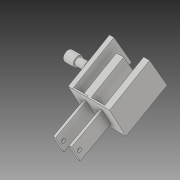
# Autodesk Inventor part: grip
Saved by Autodesk Inventor 2017 (Build 210142000, 142)
## iProperties
Created: 2021-04-21
Part Number: grip
Material: Generic
Document SubType Name: Modeling
Designer: Anthony
Density: 1 g/cm^3
Appearance: Default
Author: Anthony
Autodesk Inventor part; units mm, degrees
sketch "Sketch1" plane through (0, 0, 0) normal (1, 0, 0) x (0, 1, 0)
  line L0 (15, -38) -> (-51, -38)
  line L1 (-51, -38) -> (-51, -56)
  line L2 (-51, -56) -> (15, -56)
  line L3 (15, -38) -> (15, -56)
  arc A0 (29.5, -43.2058) -> (20.5, -58.7942) centre (25, -51) ccw
  arc A1 (33.0623, -37.0358) -> (16.9377, -64.9642) centre (25, -51) ccw
  line L4 (29.5, -43.2058) -> (39.0263, -48.7058)
  line L5 (20.5, -58.7942) -> (30.0263, -64.2942)
  line L6 (16.9377, -64.9642) -> (26.464, -70.4642)
  line L7 (33.0623, -37.0358) -> (42.5885, -42.5358)
  line L8 (42.5885, -42.5358) -> (39.0263, -48.7058)
  line L9 (30.0263, -64.2942) -> (26.464, -70.4642)
  line L10 (-51, -38) -> (-79, -38)
  line L11 (-79, -38) -> (-79, -56)
  line L12 (-51, -56) -> (-79, -56)
  dimension "d1" = 18
  constraints: 26 end point, 5 perpendicular, 4 point on circle, 3 tangent, 2 centre point, 2 horizontal, 1 coincident, 1 vertical
  measures "d1" diameter of A0
extrude "Extrusion1" add sketch "Sketch1" along normal blind 10 contours L3 A1 L2 L1 L0 | A1 L7 L8 L4 A0 L5 L9 L6 L2 L3 | L3 L2 A1
thicken "Thicken1" operation add thickness 5 both sides no extend neighbours yes toward (0, 0.8660254, -0.5) faces at (3.3333, 28.8389, -66.3509)
thicken "Thicken2" operation add thickness 5 both sides no extend neighbours yes toward (0, 0.8660254, -0.5) faces at (3.3333, 41.4011, -44.5924)
thicken "Thicken3" operation add thickness 200 both sides no extend neighbours yes toward (0, -1, 0) faces at (3.3333, -51, -44)
thicken "Thicken4" operation add thickness 30 both sides no extend neighbours yes toward (-1, 0, 0) faces at (0, -75.4432, -44)
sketch "Sketch2" plane through (10, 0, 0) normal (1, 0, 0) x (0, 0, -1)
  arc A0 (37.0358, 33.0623) -> (38.3509, 15) centre (51, 25) ccw projected
  line L0 (56, 10) -> (38.3509, 15)
  line L1 (38.3509, 15) -> (23, -17)
  line L2 (23, -17) -> (9, -332)
  line L3 (9, -332) -> (100, -328)
  line L4 (100, -328) -> (71, -47)
  line L5 (71, -47) -> (56, 10)
  point P0 (0, 0)
  constraints: 12 end point
extrude "Extrusion2" cut sketch "Sketch2" against normal blind 100
sketch "Sketch3" plane through (10, 0, 0) normal (1, 0, 0) x (0, 0, -1)
  line L0 (56, 10) -> (152, -151)
  line L1 (152, -151) -> (131, -151)
  line L2 (38.3509, 15) -> (56, 10) projected
  line L3 (131, -151) -> (38.3509, 15)
  point P0 (0, 0)
  constraints: 6 end point, 1 horizontal
extrude "Extrusion3" add sketch "Sketch3" against normal blind 40
thicken "Thicken5" operation add thickness 100 both sides no extend neighbours yes toward (0, -1, 0) faces at (-3.3333, -151, -145)
sketch "Sketch4" plane through (10, 0, 0) normal (1, 0, 0) x (0, 0, -1)
  line L0 (29, -65) -> (197, -65)
  line L1 (197, -65) -> (243, -262)
  line L2 (243, -262) -> (173, -278.3452)
  line L3 (173, -278.3452) -> (29, -65)
  point P0 (0, 0)
  constraints: 8 end point, 1 horizontal, 1 perpendicular
extrude "Extrusion4" cut sketch "Sketch4" against normal blind 40
thicken "Thicken6" operation add thickness 40 both sides no extend neighbours yes toward (1, 0, 0) faces at (10, 14.7562, -38.117)
thicken "Thicken7" operation add thickness 5 both sides no extend neighbours yes toward (0, -0.5, -0.8660254) faces at (-16.6667, 26.1753, -70.2976) (-3.3333, 10.1872, -57.3703) (-3.3333, -15.1835, -71.0162)
ref_plane "Work Plane1" through (10, -65, -83.0011) normal (1, 0, 0) x (0, 0, -1)
sketch "Sketch6" plane through (10, -65, -83.0011) normal (1, 0, 0) x (0, 0, -1)
  line L0 (23.5408, 0) -> (0, 0) projected
  line L1 (23.5408, 0) -> (65, -73)
  line L2 (65, -73) -> (86.5815, -111)
  line L3 (0, 0) -> (-44.6502, 80) projected
  line L4 (0, 0) -> (59, -111)
  line L5 (59, -111) -> (86.5815, -111)
  point P0 (-83.0011, 65)
  constraints: 8 end point, 1 horizontal, 1 point on line
extrude "Extrusion6" add sketch "Sketch6" along normal mid plane 40
thicken "Thicken8" operation add thickness 100 both sides no extend neighbours yes toward (0, -1, 0) faces at (3.3333, -176, -151.1949)
thicken "Thicken9" operation add thickness 20 both sides no extend neighbours yes toward (0, 0.8660254, -0.5) faces at (-16.6667, 45.7312, -47.0924)
thicken "Thicken10" operation add thickness 20 both sides no extend neighbours yes toward (0, 0.8660254, -0.5) faces at (-3.3333, 32.3357, -70.2943)
sketch "Sketch7" plane through (30, -65, -83.0011) normal (1, 0, 0) x (0, 0, -1)
  line L0 (112.1532, -211) -> (143.3749, -211) projected
  line L1 (23.5408, 0) -> (143.3749, -211) projected
  line L2 (143.3749, -211) -> (130, -187.4499)
  line L3 (130, -187.4499) -> (99.6355, -187.4499)
  line L4 (0, 0) -> (112.1532, -211) projected
  line L5 (112.1532, -211) -> (99.6355, -187.4499)
  point P0 (-83.0011, 65)
  constraints: 6 end point, 2 point on line, 1 collinear, 1 horizontal
extrude "Extrusion7" add sketch "Sketch7" against normal blind 400
thicken "Thicken12" operation add thickness 65 both sides no extend neighbours yes toward (1, 0, 0) faces at (-370, -268.15, -211.5104)
sketch "Sketch8" plane through (-305, -276, -226.376) normal (-1, 0, 0) x (0, 0, 1)
  line L0 (43.7393, 23.5501) -> (13.3749, 23.5501) projected
  line L1 (43.7393, 23.5501) -> (20.991, 36.7127)
  line L2 (13.3749, 23.5501) -> (43.7393, 23.5501) projected
  line L3 (20.991, 36.7127) -> (13.3749, 23.5501)
  point P0 (226.376, 276)
  constraints: 4 end point, 1 perpendicular
extrude "Extrusion8" add sketch "Sketch8" against normal blind 300
sketch "Sketch9" plane through (-305, -239.2873, -205.385) normal (0, 0.8655505, 0.5008216) x (1, 0, 0)
  line L0 (0, -0.2177) -> (0, -27.2417) projected
  line L1 (0, -0.2177) -> (0, -27.2417)
  line L2 (0, -27.2417) -> (29, -27.2417)
  line L3 (0, -27.2417) -> (335, -27.2417) projected
  line L4 (0, -0.2177) -> (29, -0.2177)
  line L5 (0, -0.2177) -> (335, -0.2177) projected
  line L6 (29, -27.2417) -> (29, -0.2177)
  point P0 (305, -57.9308)
  constraints: 8 end point, 2 point on line, 1 perpendicular, 1 vertical
extrude "Extrusion9" add sketch "Sketch9" along normal blind 70
thicken "Thicken13" operation add thickness 15 both sides no extend neighbours yes toward (0, -0.8655505, -0.5008216) faces at (-295.3333, -187.8307, -154.5452)
thicken "Thicken14" operation add thickness 7 both sides no extend neighbours yes toward (0, -0.8655505, -0.5008216) faces at (-295.3333, -200.8139, -162.0576)
sketch "Sketch10" plane through (-276, -239.3964, -205.1965) normal (0, 0.5008216, -0.8655505) x (-1, 0, 0)
  line L0 (0, 48) -> (29, 48) projected
  line L1 (0, 48) -> (-35, 48)
  line L2 (-35, 48) -> (-35, 81)
  line L3 (-35, 81) -> (-35, 106)
  line L4 (29, 48) -> (29, 121)
  line L5 (-35, 106) -> (-35, 138)
  line L6 (-35, 138) -> (-45, 138)
  line L7 (-45, 138) -> (-45, 41)
  line L8 (-45, 41) -> (29, 41)
  line L9 (29, 0) -> (29, 48) projected
  line L10 (29, 41) -> (29, 48)
  line L11 (29, 48) -> (29, 41)
  line L12 (29, 121) -> (29, 141)
  line L13 (29, 141) -> (38, 141)
  line L14 (38, 141) -> (38, 41)
  line L15 (38, 41) -> (29, 41)
  line L16 (29, 81) -> (0, 81)
  line L17 (0, 81) -> (0, 48)
  point P0 (-276, 309.9765)
  dimension "d49" = 35
  constraints: 32 end point, 8 perpendicular, 4 vertical, 2 horizontal, 2 point on line, 1 collinear
  measures "d49" distance of L0.start L1.end
extrude "Extrusion10" add sketch "Sketch10" along normal blind 70 contours L0 L9 L8 L7 L6 L5 L3 L2 L1 | L4 L12 L13 L14 L15 L9
sketch "Sketch12" plane through (-276, -204.3389, -265.785) normal (0, 0.5008216, -0.8655505) x (-1, 0, 0)
  line L0 (29, 48) -> (0, 48) projected
  line L1 (14.5, 48) -> (14.5, 123)
  line L2 (14.5, 123) -> (-8, 123)
  line L3 (-8, 123) -> (-8, 48)
  line L4 (-8, 48) -> (14.5, 48)
  point P0 (-276, 309.9765)
  constraints: 8 end point, 2 perpendicular, 1 collinear, 1 midpoint, 1 vertical
extrude "Extrusion11" add sketch "Sketch12" against normal blind 70
thicken "Thicken15" operation add thickness 2 both sides no extend neighbours yes toward (-1, 0, 0) faces at (-268, -142.8866, -176.3122)
thicken "Thicken16" operation add thickness 2 both sides no extend neighbours yes toward (1, 0, 0) faces at (-290.5, -142.8866, -176.3122)
thicken "Thicken17" operation add thickness 4 both sides no extend neighbours yes toward (1, 0, 0) faces at (-288.5, -142.8866, -176.3122)
thicken "Thicken18" operation add thickness 2 both sides no extend neighbours yes toward (-1, 0, 0) faces at (-241, -160.1976, -186.3286)
ref_plane "Work Plane2" through (-137.5, -65, -83.0011) normal (1, 0, 0) x (0, 0, -1)
sketch "Sketch13" plane through (-137.5, -65, -83.0011) normal (1, 0, 0) x (0, 0, -1)
  line L0 (143.3749, -211) -> (112.1532, -211) projected
  line L1 (130, -187.4499) -> (143.3749, -211) projected
  line L2 (143.3749, -211) -> (14, -211)
  line L3 (14, -211) -> (14, -187.4499)
  line L4 (14, -187.4499) -> (130, -187.4499)
  point P0 (-83.0011, 65)
  constraints: 6 end point, 2 perpendicular, 1 point on line
extrude "Extrusion12" add sketch "Sketch13" along normal mid plane 30
thicken "Thicken19" operation add thickness 150 both sides no extend neighbours yes toward (0, 0, 1) faces at (-142.5, -260.3, -97.0011)
thicken "Thicken20" operation add thickness 20 both sides no extend neighbours yes toward (0, 0, -1) faces at (-142.5, -260.3, 52.9989)
sketch "Sketch14" plane through (-152.5, -276, 32.9989) normal (0, 0, 1) x (1, 0, 0)
  line L0 (30, 23.5501) -> (30, 0) projected
  line L1 (0, 23.5501) -> (30, 23.5501) projected
  line L2 (0, 0) -> (30, 0) projected
  line L3 (0, 0) -> (0, 23.5501) projected
  circle A0 centre (15, 11.775) radius 8
  point P0 (152.5, 276)
  constraints: 1 centre point
extrude "Extrusion13" add sketch "Sketch14" along normal blind 70 contours A0
thicken "Thicken21" operation add thickness 30 both sides no extend neighbours yes toward (0, 0, -1) faces at (-134.9108, -264.8631, 102.9989)
sketch "Sketch15" plane through (-122.5, -65, -83.0011) normal (1, 0, 0) x (0, 0, -1)
  arc A0 (-202, -264) -> (-180, -132) centre (-216.7127, -193.7146) ccw
  arc A1 (-204.0725, -254.0995) -> (-185.1714, -140.6932) centre (-216.7127, -193.7146) ccw
  arc A2 (-200.0254, -273.433) -> (-175.0728, -123.7173) centre (-216.7127, -193.7146) ccw
  line L0 (-175.0728, -123.7173) -> (-185.1714, -140.6932)
  line L1 (-204.0725, -254.0995) -> (-200.0254, -273.433)
  point P0 (-83.0011, 65)
  constraints: 6 point on circle, 4 end point, 3 centre point
extrude "Extrusion14" add sketch "Sketch15" against normal blind 30
sketch "Sketch16" plane through (-122.5, -65, -83.0011) normal (1, 0, 0) x (0, 0, -1)
  point P0 (-83.0011, 65)
ref_plane "Work Plane3" through (-137.5, -65, -83.0011) normal (1, 0, 0) x (0, 0, -1)
sketch "Sketch17" plane through (-137.5, -65, -83.0011) normal (1, 0, 0) x (0, 0, -1)
  arc A0 (-204.0725, -254.0995) -> (-185.1714, -140.6932) centre (-216.7127, -193.7146) ccw projected
  arc A1 (-200.5833, -270.7677) -> (-176.465, -126.0576) centre (-216.7127, -193.7146) ccw
  line L0 (-176.465, -126.0576) -> (-223, -140.6932)
  line L1 (-223, -140.6932) -> (-219, -249)
  line L2 (-219, -249) -> (-200.5833, -270.7677)
  point P0 (-83.0011, 65)
  constraints: 6 end point, 2 point on circle, 1 centre point
extrude "Extrusion15" cut sketch "Sketch17" against normal blind 14
sketch "Sketch18" plane through (-122.5, -65, -83.0011) normal (1, 0, 0) x (0, 0, -1)
  point P0 (-83.0011, 65)
ref_plane "Work Plane4" through (-124.5, -65, -83.0011) normal (1, 0, 0) x (0, 0, -1)
sketch "Sketch19" plane through (-124.5, -65, -83.0011) normal (1, 0, 0) x (0, 0, -1)
  arc A0 (-200.0254, -273.433) -> (-175.0728, -123.7173) centre (-216.7127, -193.7146) ccw projected
  arc A1 (-200.6398, -270.4982) -> (-176.6058, -126.2942) centre (-216.7127, -193.7146) ccw
  line L0 (-176.6058, -126.2942) -> (-213.3412, -154.8678)
  line L1 (-213.3412, -154.8678) -> (-216.7127, -283)
  line L2 (-216.7127, -283) -> (-200.6398, -270.4982)
  point P0 (-83.0011, 65)
  constraints: 6 end point, 2 point on circle, 1 centre point, 1 parallel
extrude "Extrusion16" cut sketch "Sketch19" against normal blind 14
thicken "Thicken22" operation add thickness 150 both sides no extend neighbours yes toward (1, 0, 0) faces at (-122.5, -268.15, -114.9306)
thicken "Thicken23" operation add thickness 150 both sides no extend neighbours yes toward (1, 0, 0) faces at (-152.5, -268.15, -114.9306)
thicken "Thicken24" operation add thickness 150 both sides no extend neighbours yes toward (1, 0, 0) faces at (-122.5, -266.9722, 59.5019)
thicken "Thicken25" operation add thickness 150 both sides no extend neighbours yes toward (1, 0, 0) faces at (-152.5, -266.9722, 59.5019)
sketch "Sketch20" plane through (-137.5, -264.225, 32.9989) normal (0, 0, -1) x (-1, 0, 0)
  circle A0 centre (0, 0) radius 10.0499
  point P0 (-137.5, 264.225)
  constraints: 1 centre point, 1 other
extrude "Extrusion17" cut sketch "Sketch20" against normal blind 40
sketch "Sketch21" plane through (27.5, -276, 32.9989) normal (0, 0, 1) x (1, 0, 0)
  circle A0 centre (-13, 11) radius 8.9443
  point P0 (-27.5, 276)
  constraints: 1 centre point
extrude "Extrusion18" add sketch "Sketch21" along normal blind 40
thicken "Thicken26" operation add thickness 3 both sides no extend neighbours yes toward (0, -0.5353442, -0.844634) faces at (17.5, -302.3163, 64.9194) (7.5, -200.0346, 98.8042) (7.5, -331.9885, 118.3734) (17.5, -291.7419, 81.603)
thicken "Thicken27" operation add thickness 3 both sides no extend neighbours yes toward (-1, 0, 0) faces at (-2.5, -241.3228, 60.0882)
sketch "Sketch23" plane through (30, -65, -83.0011) normal (1, 0, 0) x (0, 0, -1)
  line L0 (143.3749, -211) -> (23.5408, 0) projected
  line L1 (112.1532, -211) -> (143.3749, -211) projected
  line L2 (0, 0) -> (112.1532, -211) projected
  line L3 (112.1532, -211) -> (227, -459)
  line L4 (227, -459) -> (284.2225, -459)
  line L5 (284.2225, -459) -> (143.3749, -211)
  point P0 (-83.0011, 65)
  constraints: 6 end point, 1 horizontal
extrude "Extrusion19" add sketch "Sketch23" against normal blind 50
sketch "Sketch24" plane through (30.5, -258.7146, 133.7116) normal (1, 0, 0) x (0, -0.164399, -0.9863939)
  point P0 (89.3599, 277.1765)
ref_plane "Work Plane5" through (28.5, -258.7146, 133.7116) normal (1, 0, 0) x (0, -0.164399, -0.9863939)
sketch "Sketch25" plane through (28.5, -258.7146, 133.7116) normal (1, 0, 0) x (0, -0.164399, -0.9863939)
  arc A0 (29.5658, -75.8904) -> (29.5658, 75.8904) centre (0, 0) ccw projected
  arc A1 (28.9727, -74.3679) -> (28.9727, 74.3679) centre (0, 0) ccw
  line L0 (28.9727, 74.3679) -> (10, 52)
  line L1 (10, 52) -> (7, -23)
  line L2 (7, -23) -> (7, -70)
  line L3 (7, -70) -> (28.9727, -74.3679)
  point P0 (89.3599, 277.1765)
  constraints: 8 end point, 2 point on circle, 1 centre point, 1 vertical
extrude "Extrusion20" cut sketch "Sketch25" against normal blind 31
sketch "Sketch26" plane through (-10, -65, -83.0011) normal (0, -0.4693491, 0.8830127) x (1, 0, 0)
  line L0 (-323, -166) -> (-187, -166)
  line L1 (-221, -167.8541) -> (-304, -167.8541) projected
  line L2 (-187, -166) -> (-176, 142)
  line L3 (-176, 142) -> (163, 177)
  line L4 (163, 177) -> (104, -166)
  line L5 (104, -166) -> (180, -544)
  line L6 (180, -544) -> (-44, -703)
  line L7 (-44, -703) -> (-203.3393, -623.5)
  line L8 (-203.3393, -623.5) -> (-196.1783, -422.9935)
  line L9 (-196.1783, -422.9935) -> (-455, -378.4732)
  line L10 (-455, -378.4732) -> (-323, -166)
  point P0 (10, 96.3523)
  constraints: 20 end point, 3 point on line, 1 parallel, 1 perpendicular
extrude "Extrusion21" cut sketch "Sketch26" along normal mid plane 1000
sketch "Sketch27" plane through (-305, -211.3842, -157.7664) normal (0, 0.8655505, 0.5008216) x (1, 0, 0)
  line L0 (0, 27) -> (45, 27)
  line L1 (45, 27) -> (45, -17)
  line L2 (45, -17) -> (8, -14)
  line L3 (8, -14) -> (-11, 2)
  line L4 (-11, 2) -> (0, 27)
  point P0 (305, -30.6891)
  constraints: 10 end point, 1 horizontal, 1 perpendicular
extrude "Extrusion22" cut sketch "Sketch27" against normal blind 10
sketch "Sketch28" plane through (-314, -167.2455, -244.3222) normal (0, -0.8830127, -0.4693491) x (1, 0, 0)
  line L0 (83, 0) -> (0, 0) projected
  line L1 (83, 70.0454) -> (83, 0) projected
  line L2 (0, 0) -> (0, 70.0454) projected
  point P0 (314, 137.2431)
sketch "Sketch29" plane through (-314, -167.2455, -244.3222) normal (0, -0.8830127, -0.4693491) x (1, 0, 0)
  line L0 (60, 15) -> (23, 15)
  line L1 (23, 15) -> (23, 52)
  line L2 (23, 52) -> (60, 52)
  line L3 (60, 52) -> (60, 15)
  point P0 (314, 137.2431)
  constraints: 8 end point, 2 parallel, 1 horizontal, 1 perpendicular
extrude "Extrusion23" add sketch "Sketch29" along normal blind 70
sketch "Sketch30" plane through (-314, -229.0564, -277.1766) normal (0, -0.8830127, -0.4693491) x (1, 0, 0)
  line L0 (23, 15) -> (60, 15) projected
  line L1 (23, 15) -> (60, 15) projected
  line L2 (60, 15) -> (60, 52) projected
  line L3 (60, 52) -> (23, 52) projected
  line L4 (23, 52) -> (23, 15) projected
  line L5 (55, 15) -> (55, 52)
  line L6 (28, 15) -> (28, 52)
  point P0 (314, 137.2431)
  constraints: 4 end point, 4 point on line, 2 perpendicular
extrude "Extrusion24" cut sketch "Sketch30" against normal blind 70 contours L6 L3 L5 L0
sketch "Sketch31" plane through (-254, -191.6516, -198.4055) normal (1, 0, 0) x (0, 0.4693491, -0.8830127)
  circle A0 centre (19, -62) radius 4.1231
  point P0 (-85.2431, 262.3523)
  constraints: 1 centre point
extrude "Extrusion25" cut sketch "Sketch31" against normal blind 70
sketch "Sketch32" plane through (-231, -119.9504, -136.0831) normal (1, 0, 0) x (0, 0.5008216, -0.8655505)
  circle A0 centre (36, -44) radius 10
  point P0 (-57.7131, 171.9765)
  constraints: 1 centre point
extrude "Extrusion26" add sketch "Sketch32" along normal blind 20
sketch "Sketch33" plane through (-211, -140.0051, -189.2791) normal (1, 0, 0) x (0, 0, -1)
  circle A0 centre (0, 0) radius 10 projected
  circle A1 centre (0, 0) radius 7
  point P0 (-189.2791, 140.0051)
  constraints: 1 centre point, 1 coincident
extrude "Extrusion27" add sketch "Sketch33" along normal blind 20 contours A1
sketch "Sketch34" plane through (-191, -140.0051, -189.2791) normal (1, 0, 0) x (0, 0, -1)
  circle A0 centre (0, 0) radius 7 projected
  circle A1 centre (0, 0) radius 10
  point P0 (-189.2791, 140.0051)
  constraints: 1 centre point, 1 coincident
extrude "Extrusion28" add sketch "Sketch34" along normal blind 20 contours A0 | A1
ref_plane "Work Plane6" through (-272.473, -82.2963, -195.1692) normal (-1, 0, 0) x (0, -0.5008216, 0.8655505)
mirror "Mirror1" about plane through (-272.473, -82.2963, -195.1692) normal (-1, 0, 0) of "Extrusion27", "Extrusion26", "Extrusion28"
sketch "Sketch35" plane through (-171, -140.0051, -189.2791) normal (1, 0, 0) x (0, 0, -1)
  circle A0 centre (0, 0) radius 18.2483
  point P0 (-189.2791, 140.0051)
  constraints: 1 centre point
extrude "Extrusion29" cut sketch "Sketch35" against normal blind 60
body "Solid1"
